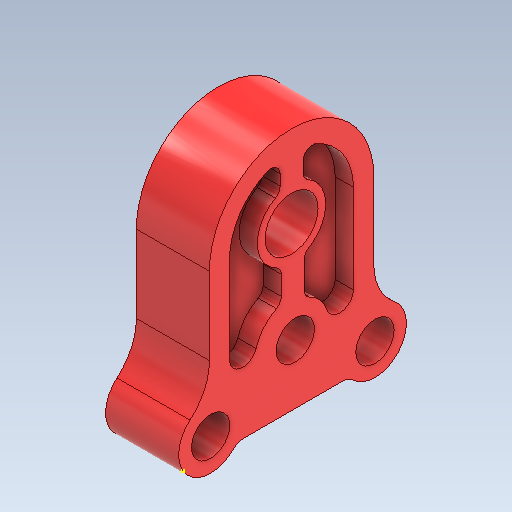
# Autodesk Inventor part: hw1
Saved by Autodesk Inventor 2021 (Build 250183000, 183)
## iProperties
Created: 2022-04-30
Part Number: hw1
Material: Generic
Document SubType Name: Modeling
Designer: authe
Density: 1 g/cm^3
Appearance: Light Red
Author: authe
Autodesk Inventor part; units mm, degrees
ref_plane "YZ Plane" through (0, 0, 0) normal (1, 0, 0) x (0, 1, 0)
ref_plane "XZ Plane" through (0, 0, 0) normal (0, 1, 0) x (-1, 0, 0)
ref_plane "XY Plane" through (0, 0, 0) normal (0, 0, 1) x (1, 0, 0)
sketch "Sketch1" plane through (0, 0, 0) normal (1, 0, 0) x (0, 1, 0)
  arc A0 (176.1097, -208.7052) -> (175.3048, -28.7073) centre (175.5363, -118.707) ccw
  line L0 (175.3048, -28.7073) -> (90.5303, -28.7073)
  line L1 (-1.9186, -65.845) -> (-1.9186, -175.1547)
  line L2 (92.0444, -208.7052) -> (176.1097, -208.7052)
  arc A1 (44.7113, -7.4451) -> (-6.4479, -55.1041) centre (17.9836, -30.0422) ccw
  arc A2 (-6.3181, -185.8489) -> (45.0423, -231.4117) centre (18.1097, -210.0421) ccw
  line L3 (175.7375, -50.7073) -> (78.1247, -50.7073)
  line L4 (133.0218, -107.5228) -> (111.9726, -107.5228)
  line L5 (105.0926, -132.5228) -> (134.6019, -132.5228)
  arc A3 (208.5623, -100.9438) -> (141.9722, -101.9826) centre (175.5363, -118.707) ccw
  arc A4 (103.0885, -102.1131) -> (76.4229, -79.7842) centre (63.1097, -122.7698) ccw
  arc A5 (74.6044, -157.3047) -> (96.0441, -138.2655) centre (63.1097, -122.7698) ccw
  circle A6 centre (63.1097, -122.7698) radius 21
  circle A7 centre (17.9836, -30.0422) radius 21
  circle A8 centre (18.1097, -210.0421) radius 21
  arc A9 (44.7113, -7.4451) -> (90.5303, -28.7073) centre (90.5303, 31.2927) ccw
  arc A10 (92.0444, -208.7052) -> (45.0423, -231.4117) centre (92.0444, -268.7052) ccw
  arc A11 (-1.9186, -65.845) -> (-6.4479, -55.1041) centre (-16.9186, -65.845) ccw
  arc A12 (-6.3181, -185.8489) -> (-1.9186, -175.1547) centre (-17.1159, -175.1547) ccw
  arc A13 (78.1247, -50.7073) -> (76.4229, -79.7842) centre (80.8606, -65.4557) ccw
  arc A14 (74.6044, -157.3047) -> (78.6837, -186.5226) centre (79.3415, -171.5371) ccw
  circle A15 centre (175.5363, -118.707) radius 29
  arc A16 (133.0218, -107.5228) -> (141.9722, -101.9826) centre (133.0218, -97.5228) ccw
  arc A17 (143.2454, -137.4939) -> (134.6019, -132.5228) centre (134.6019, -142.5228) ccw
  arc A18 (103.0885, -102.1131) -> (111.9726, -107.5228) centre (111.9726, -97.5228) ccw
  arc A19 (105.0926, -132.5228) -> (96.0441, -138.2655) centre (105.0926, -142.5228) ccw
  line L6 (217.3693, -106.207) -> (225.3783, -106.207)
  line L7 (225.3783, -106.207) -> (229.2504, -106.207)
  line L8 (225.1161, -131.2646) -> (228.7337, -131.2481)
  line L9 (228.7337, -131.2481) -> (217.1089, -131.3029)
  arc A20 (217.1089, -131.3029) -> (208.3269, -136.6074) centre (217.156, -141.3028) ccw
  arc A21 (208.5623, -100.9438) -> (217.3693, -106.207) centre (217.3693, -96.207) ccw
  line L10 (119.8472, -132.5228) -> (119.8472, -186.8276)
  arc A22 (176.0639, -186.5226) -> (238.0141, -145.0843) centre (175.5363, -118.707) ccw
  arc A23 (143.2454, -137.4939) -> (208.3269, -136.6074) centre (175.5363, -118.707) ccw
  line L11 (176.0639, -186.5226) -> (78.6837, -186.5226)
  arc A24 (238.2111, -92.3277) -> (175.7375, -50.7073) centre (175.5363, -118.707) ccw
  line L12 (229.2504, -106.207) -> (228.9942, -106.207)
  arc A25 (228.9942, -106.207) -> (238.2111, -92.3277) centre (228.9942, -96.207) ccw
  line L13 (228.7337, -131.2481) -> (228.7379, -131.2481)
  line L14 (238.2764, -144.2509) -> (238.0141, -145.0843)
  arc A26 (238.2764, -144.2509) -> (228.7379, -131.2481) centre (228.7379, -141.2481) ccw
  point P0 (0, 0)
  point P1 (0, 0)
  point P2 (-1.9186, -182.0976)
  point P3 (139.7429, -107.5228)
  point P4 (140.8602, -132.5228)
  point P5 (105.4479, -107.5228)
  point P6 (98.1763, -132.5228)
  point P7 (-1.9186, -58.8329)
  point P8 (210.8916, -106.207)
  point P9 (242.3775, -106.207)
  dimension "d36" = 60
  dimension "d37" = 42
  dimension "d38" = 35
  dimension "d40" = 42
  dimension "d41" = 45
  dimension "d42" = 45
  dimension "d50" = 90
  dimension "d51" = 15
  dimension "d52" = 15
  dimension "d53" = 15
  dimension "d54" = 180
  dimension "d55" = 60
  dimension "d64" = 58
  dimension "d66" = 25
  dimension "d68" = 10
  dimension "d69" = 37.5
  dimension "d75" = 22
  dimension "d79" = 10
  constraints: 53 point on circle, 30 end point, 27 centre point, 24 tangent, 10 point on line, 8 coincident, 8 horizontal, 5 equal radius, 2 parallel, 1 midpoint, 1 perpendicular
  measures "d36" radius of A9
  measures "d37" diameter of A7
  measures "d38" radius of A1
  measures "d40" diameter of A6
  measures "d41" radius of A4
  measures "d42" horizontal distance of A2.centre A6.centre
  measures "d50" radius of A0
  measures "d51" radius of A13
  measures "d52" radius of A14
  measures "d53" radius of A11
  measures "d54" distance of A2.centre A1.centre
  measures "d55" radius of A10
  measures "d64" diameter of A15
  measures "d66" distance between parallel lines of L5 L4
  measures "d68" radius of A16
  measures "d69" radius of A3
  measures "d75" distance between parallel lines of L0 L3
  measures "d79" radius of A25
extrude "Extrusion1" add sketch "Sketch1" along normal blind 40 and the other way blind 40
sketch "Sketch2" plane through (40, 0, 0) normal (1, 0, 0) x (0, 0, -1)
  point P0 (0, 0)
extrude "Extrusion2" add sketch "Sketch1" along normal blind 20 and the other way blind 20 contours A24 A25 L7 L6 A21 A3 A16 L4 A18 A4 A13 L3 | L5 L10 L11 A14 A5 A19 | L5 A17 A23 A20 L9 L8 L13 A26 L14 A22 L11 L10
body "Solid1"
